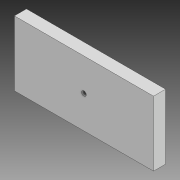
# Autodesk Inventor part: CamBracket
Saved by Autodesk Inventor 2020 (Build 240168000, 168)
## iProperties
Created: 2021-03-19
Part Number: CamBracket
Material: Generic
Document SubType Name: Modeling
Designer: DDeGo
Density: 1 g/cm^3
Appearance: Default
Author: DDeGo
Autodesk Inventor part; units mm, degrees
ref_plane "YZ Plane" through (0, 0, 0) normal (1, 0, 0) x (0, 1, 0)
ref_plane "XZ Plane" through (0, 0, 0) normal (0, 1, 0) x (-1, 0, 0)
ref_plane "XY Plane" through (0, 0, 0) normal (0, 0, 1) x (1, 0, 0)
sketch "Sketch1" plane through (0, 0, 0) normal (0, 0, 1) x (1, 0, 0)
  circle A0 centre (0, 0) radius 25
  line L0 (-75, -35) -> (75, -35)
  line L1 (75, -35) -> (75, 35)
  line L2 (75, 35) -> (-75, 35)
  line L3 (-75, 35) -> (-75, -35)
  line L4 (-75, -35) -> (75, 35) construction
  line L5 (75, -35) -> (-75, 35) construction
  dimension "d0" = 50
  dimension "d2" = 70
  dimension "d3" = 150
  constraints: 12 end point, 2 midpoint, 2 parallel, 1 centre point, 1 coincident, 1 horizontal, 1 perpendicular
  measures "d0" diameter of A0
  measures "d2" distance of L0.end L1.end
  measures "d3" distance of L0.start L0.end
extrude "Extrusion1" add sketch "Sketch1" along normal blind 10
sketch "Sketch3" plane through (75, -35, 0) normal (1, 0, 0) x (0, 0, -1)
  line L0 (-90, 0) -> (-90, 70) projected
  line L1 (-90, 35) -> (-50, 35) construction
  circle A0 centre (-50, 35) radius 25
  point P0 (0, 35)
  dimension "d10" = 50
  dimension "d11" = 40
  constraints: 2 end point, 1 centre point, 1 coincident, 1 horizontal, 1 midpoint
  measures "d10" diameter of A0
  measures "d11" distance of L1.start L1.end
extrude "Extrusion3" cut sketch "Sketch3" against normal through all
sketch "Sketch4" plane through (0, 0, 10) normal (0, 0, 1) x (1, 0, 0)
  line L0 (-75, 35) -> (-75, -35) projected
  line L1 (-75, -35) -> (75, -35) projected
  line L2 (75, -35) -> (75, 35) projected
  line L3 (75, 35) -> (-75, 35) projected
  circle A0 centre (0, 0) radius 25 construction
  circle A1 centre (0, 0) radius 2.5
  dimension "d14" = 5
  constraints: 1 centre point, 1 coincident
  measures "d14" diameter of A1
extrude "Extrusion4" add sketch "Sketch4" along normal blind 3
body "Solid1"
